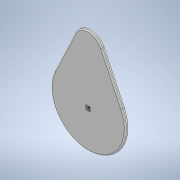
# Autodesk Inventor part: 4.2 Part D
Saved by Autodesk Inventor 2020 (Build 240168000, 168)
## iProperties
Created: 2020-01-07
Part Number: 4.2 Part D
Material: Generic
Document SubType Name: Modeling
Designer: cks4a449
Density: 1 g/cm^3
Appearance: Default
Author: cks4a449
Autodesk Inventor part; units mm, degrees
ref_plane "YZ Plane" through (0, 0, 0) normal (1, 0, 0) x (0, 1, 0)
ref_plane "XZ Plane" through (0, 0, 0) normal (0, 1, 0) x (-1, 0, 0)
ref_plane "XY Plane" through (0, 0, 0) normal (0, 0, 1) x (1, 0, 0)
sketch "Sketch2" plane through (0, 0, 0) normal (0, 0, 1) x (1, 0, 0)
  arc A0 (-28.6864, 13.6071) -> (28.6864, 13.6071) centre (0, 0) ccw
  arc A1 (11.4746, 49.8929) -> (-11.4746, 49.8929) centre (0, 44.45) ccw
  line L0 (-28.6864, 13.6071) -> (-11.4746, 49.8929)
  line L1 (11.4746, 49.8929) -> (28.6864, 13.6071)
  line L2 (-1.5875, -1.5875) -> (-1.5875, 1.5875)
  line L3 (-1.5875, 1.5875) -> (1.5875, 1.5875)
  line L4 (1.5875, 1.5875) -> (1.5875, -1.5875)
  line L5 (1.5875, -1.5875) -> (-1.5875, -1.5875)
  line L6 (-1.5875, -1.5875) -> (1.5875, 1.5875) construction
  line L7 (-1.5875, 1.5875) -> (1.5875, -1.5875) construction
  dimension "d16" = 63.5
  dimension "d18" = 25.4
  dimension "d19" = 44.45
  dimension "d22" = 3.175
  dimension "d23" = 3.175
  constraints: 16 end point, 4 point on circle, 4 tangent, 2 centre point, 2 midpoint, 2 parallel, 1 coincident, 1 perpendicular, 1 vertical
  measures "d16" diameter of A0
  measures "d18" diameter of A1
  measures "d19" distance of point (0, 0) A1.centre
  measures "d22" distance of L2.start L2.end
  measures "d23" distance of L2.end L3.end
extrude "Extrusion3" add sketch "Sketch2" along normal blind 3.175
fillet "Fillet3" radius 1.016 8 edges at (0, 57.15, 3.175) (-20.0805, 31.75, 3.175) (0, -31.75, 3.175) (20.0805, 31.75, 3.175) (0, 57.15, 0) (-20.0805, 31.75, 0) (0, -31.75, 0) (20.0805, 31.75, 0)
chamfer "Chamfer1" distance 0.254 angle 45 8 edges at (1.5875, 0, 3.175) (0, -1.5875, 3.175) (-1.5875, 0, 3.175) (0, 1.5875, 3.175) (0, -1.5875, 0) (-1.5875, 0, 0) (0, 1.5875, 0) (1.5875, 0, 0)
body "Solid3"
